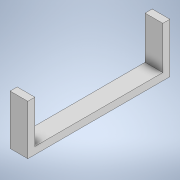
# Autodesk Inventor part: guitar bridge
Saved by Autodesk Inventor 2021 (Build 250183000, 183)
## iProperties
Created: 2021-07-03
Part Number: guitar bridge
Material: Generic
Document SubType Name: Modeling
Designer: Aditya Nellikeri
Density: 1 g/cm^3
Appearance: Default
Author: Aditya Nellikeri
Autodesk Inventor part; units mm, degrees
ref_plane "YZ Plane" through (0, 0, 0) normal (1, 0, 0) x (0, 1, 0)
ref_plane "XZ Plane" through (0, 0, 0) normal (0, 1, 0) x (-1, 0, 0)
ref_plane "XY Plane" through (0, 0, 0) normal (0, 0, 1) x (1, 0, 0)
sketch "Sketch1" plane through (0, 0, 0) normal (0, 1, 0) x (-1, 0, 0)
  line L0 (0, 0) -> (-63.5, 0)
  line L1 (-63.5, 0) -> (-63.5, -508)
  line L2 (-63.5, -508) -> (0, -508)
  line L3 (0, -508) -> (0, 0)
  dimension "d0" = 63.5
  dimension "d1" = 508
  constraints: 8 end point, 2 parallel, 1 horizontal, 1 perpendicular
  measures "d0" distance of L2.end L1.end
  measures "d1" distance of L0.end L1.end
extrude "Extrusion1" add sketch "Sketch1" along normal blind 25.4
sketch "Sketch2" plane through (0, 25.4, 0) normal (0, 1, 0) x (1, 0, 0)
  line L0 (0, 508) -> (0, 0) projected
  line L1 (63.5, 0) -> (63.5, 508) projected
  line L2 (0, 0) -> (63.5, 0)
  line L3 (63.5, 0) -> (63.5, 25.4)
  line L4 (63.5, 25.4) -> (0, 25.4)
  line L5 (0, 25.4) -> (0, 0)
  line L6 (0, 508) -> (63.5, 508)
  line L7 (63.5, 508) -> (63.5, 482.6)
  line L8 (63.5, 482.6) -> (0, 482.6)
  line L9 (0, 482.6) -> (0, 508)
  dimension "d4" = 25.4
  dimension "d5" = 25.4
  constraints: 16 end point, 4 parallel, 3 point on line, 2 horizontal, 2 perpendicular
  measures "d4" distance of L3.end L2.end
  measures "d5" distance of L6.end L7.end
extrude "Extrusion2" add sketch "Sketch2" along normal blind 152.4 contours L6 L1 L8 L0 | L4 L1 L2 L0
sketch "Sketch3" plane through (0, 0, 0) normal (0, -1, 0) x (1, 0, 0)
  line L0 (0, -482.6) -> (0, -25.4) projected
  line L1 (0, -406.4) -> (5.08, -406.4)
  line L2 (5.08, -406.4) -> (5.08, -101.6)
  line L3 (5.08, -101.6) -> (0, -101.6)
  line L4 (0, -101.6) -> (0, -406.4)
  point P0 (0, 0)
  dimension "d8" = 5.08
  dimension "d9" = 304.8
  constraints: 8 end point, 2 parallel, 1 horizontal, 1 perpendicular, 1 point on line
  measures "d8" distance of L3.end L2.end
  measures "d9" distance of L2.end L1.end
extrude "Extrusion3" add sketch "Sketch3" along normal blind 38.1
sketch "Sketch4" plane through (0, 0, 0) normal (-1, 0, 0) x (0, 0, 1)
  line L0 (-192.6336, -30.2006) -> (-204.6224, -30.2006)
  line L1 (-204.6224, -30.2006) -> (-204.6224, -7.8994)
  line L2 (-204.6224, -7.8994) -> (-192.6336, -7.8994)
  line L3 (-192.6336, -7.8994) -> (-192.6336, -30.2006)
  line L4 (-214.7824, -30.2006) -> (-226.7712, -30.2006)
  line L5 (-226.7712, -30.2006) -> (-226.7712, -7.8994)
  line L6 (-226.7712, -7.8994) -> (-214.7824, -7.8994)
  line L7 (-214.7824, -7.8994) -> (-214.7824, -30.2006)
  line L8 (-236.9312, -30.2006) -> (-248.92, -30.2006)
  line L9 (-248.92, -30.2006) -> (-248.92, -7.8994)
  line L10 (-248.92, -7.8994) -> (-236.9312, -7.8994)
  line L11 (-236.9312, -7.8994) -> (-236.9312, -30.2006)
  line L12 (-259.08, -30.2006) -> (-271.0688, -30.2006)
  line L13 (-271.0688, -30.2006) -> (-271.0688, -7.8994)
  line L14 (-271.0688, -7.8994) -> (-259.08, -7.8994)
  line L15 (-259.08, -7.8994) -> (-259.08, -30.2006)
  line L16 (-281.2288, -30.2006) -> (-293.2176, -30.2006)
  line L17 (-293.2176, -30.2006) -> (-293.2176, -7.8994)
  line L18 (-293.2176, -7.8994) -> (-281.2288, -7.8994)
  line L19 (-281.2288, -7.8994) -> (-281.2288, -30.2006)
  line L20 (-303.3776, -30.2006) -> (-315.3664, -30.2006)
  line L21 (-315.3664, -30.2006) -> (-315.3664, -7.8994)
  line L22 (-315.3664, -7.8994) -> (-303.3776, -7.8994)
  line L23 (-303.3776, -7.8994) -> (-303.3776, -30.2006)
  line L24 (-406.4, 0) -> (-406.4, -38.1) projected
  circle A0 centre (-198.628, -32.8422) radius 1.1049
  circle A1 centre (-198.628, -5.2578) radius 1.1049
  circle A2 centre (-220.7768, -32.8422) radius 1.1049
  circle A3 centre (-220.7768, -5.2578) radius 1.1049
  circle A4 centre (-242.9256, -32.8422) radius 1.1049
  circle A5 centre (-242.9256, -5.2578) radius 1.1049
  circle A6 centre (-265.0744, -32.8422) radius 1.1049
  circle A7 centre (-265.0744, -5.2578) radius 1.1049
  circle A8 centre (-287.2232, -32.8422) radius 1.1049
  circle A9 centre (-287.2232, -5.2578) radius 1.1049
  circle A10 centre (-309.372, -32.8422) radius 1.1049
  circle A11 centre (-309.372, -5.2578) radius 1.1049
  line L25 (-101.6, 0) -> (-101.6, -38.1) projected
  point P0 (0, 0)
  dimension "d12" = 11.9888
  dimension "d13" = 22.3012
  dimension "d14" = 11.9888
  dimension "d15" = 22.3012
  dimension "d16" = 11.9888
  dimension "d17" = 22.3012
  dimension "d18" = 11.9888
  dimension "d19" = 22.3012
  dimension "d20" = 11.9888
  dimension "d21" = 22.3012
  dimension "d22" = 11.9888
  dimension "d23" = 22.3012
  dimension "d24" = 10.16
  dimension "d25" = 10.16
  dimension "d26" = 10.16
  dimension "d27" = 10.16
  dimension "d28" = 10.16
  dimension "d29" = 91.0336
  dimension "d30" = 2.2098
  dimension "d31" = 2.2098
  dimension "d32" = 2.2098
  dimension "d33" = 2.2098
  dimension "d34" = 2.2098
  dimension "d35" = 2.2098
  dimension "d36" = 2.2098
  dimension "d37" = 2.2098
  dimension "d38" = 2.2098
  dimension "d39" = 2.2098
  dimension "d40" = 2.2098
  dimension "d41" = 2.2098
  dimension "d42" = 22.1488
  dimension "d43" = 97.028
  dimension "d44" = 22.1488
  dimension "d45" = 22.1488
  dimension "d46" = 22.1488
  dimension "d47" = 22.1488
  dimension "d48" = 22.1488
  dimension "d49" = 22.1488
  dimension "d50" = 22.1488
  dimension "d51" = 22.1488
  dimension "d52" = 22.1488
  dimension "d53" = 97.028
  constraints: 48 end point, 12 centre point, 12 parallel, 6 horizontal, 6 perpendicular
  measures "d12" distance of L1.end L2.end
  measures "d13" distance of L0.end L1.end
  measures "d14" distance of L5.end L7.start
  measures "d15" distance of L4.end L5.end
  measures "d16" distance of L9.end L11.start
  measures "d17" distance of L8.end L9.end
  measures "d18" distance of L13.end L15.start
  measures "d19" distance of L12.end L13.end
  measures "d20" distance of L17.end L19.start
  measures "d21" distance of L16.end L17.end
  measures "d22" distance of L21.end L23.start
  measures "d23" distance of L20.end L21.end
  measures "d24" distance between parallel lines of L7 L1
  measures "d25" distance between parallel lines of L11 L5
  measures "d26" distance between parallel lines of L15 L9
  measures "d27" distance between parallel lines of L19 L13
  measures "d28" distance between parallel lines of L23 L17
  measures "d29" distance between parallel lines of L24 L21
  measures "d30" diameter of A0
  measures "d31" diameter of A1
  measures "d32" diameter of A2
  measures "d33" diameter of A3
  measures "d34" diameter of A4
  measures "d35" diameter of A5
  measures "d36" diameter of A6
  measures "d37" diameter of A7
  measures "d38" diameter of A8
  measures "d39" diameter of A9
  measures "d40" diameter of A10
  measures "d41" diameter of A11
  measures "d42" distance of A2.centre A0.centre
  measures "d43" distance from line of A0.centre L25
  measures "d44" distance of A3.centre A1.centre
  measures "d45" distance of A4.centre A2.centre
  measures "d46" distance of A5.centre A3.centre
  measures "d47" distance of A6.centre A4.centre
  measures "d48" distance of A7.centre A5.centre
  measures "d49" distance of A8.centre A6.centre
  measures "d50" distance of A9.centre A7.centre
  measures "d51" distance of A10.centre A8.centre
  measures "d52" distance of A11.centre A9.centre
  measures "d53" distance from line of A1.centre L25
extrude "Extrusion4" cut sketch "Sketch4" against normal blind 5.08
body "Solid1"
